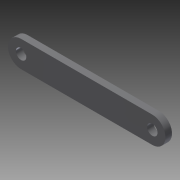
# Autodesk Inventor part: Lamp arm 2
Saved by Autodesk Inventor 2015 (Build 190159000, 159)
## iProperties
Created: 2017-04-18
Part Number: Lamp arm 2
Material: ABS Plastic
Document SubType Name: Modeling
Designer: Silas
Density: 1.06 g/cm^3
Appearance: Smooth - White
Author: Silas
Autodesk Inventor part; units mm, degrees
ref_plane "YZ Plane" through (0, 0, 0) normal (1, 0, 0) x (0, 1, 0)
ref_plane "XZ Plane" through (0, 0, 0) normal (0, 1, 0) x (-1, 0, 0)
ref_plane "XY Plane" through (0, 0, 0) normal (0, 0, 1) x (1, 0, 0)
sketch "Sketch1" plane through (0, 0, 0) normal (0, 1, 0) x (-1, 0, 0)
  line L0 (0, 0) -> (100, 0) construction
  line L1 (0, -10) -> (100, -10)
  line L2 (100, 10) -> (0, 10)
  arc A0 (0, 10) -> (0, -10) centre (0, 0) ccw
  arc A1 (100, -10) -> (100, 10) centre (100, 0) ccw
  circle A2 centre (0, 0) radius 4
  circle A3 centre (100, 0) radius 4
  point P0 (50, 0)
  dimension "d0" = 100
  dimension "d1" = 20
  dimension "d2" = 8
  dimension "d3" = 8
  constraints: 8 end point, 4 centre point, 4 point on circle, 4 tangent, 2 coincident, 1 horizontal, 1 midpoint, 1 parallel
  measures "d0" distance of L0.start L0.end
  measures "d1" diameter of A1
  measures "d2" diameter of A2
  measures "d3" diameter of A3
extrude "Extrusion1" add sketch "Sketch1" along normal blind 5
body "Solid1"
